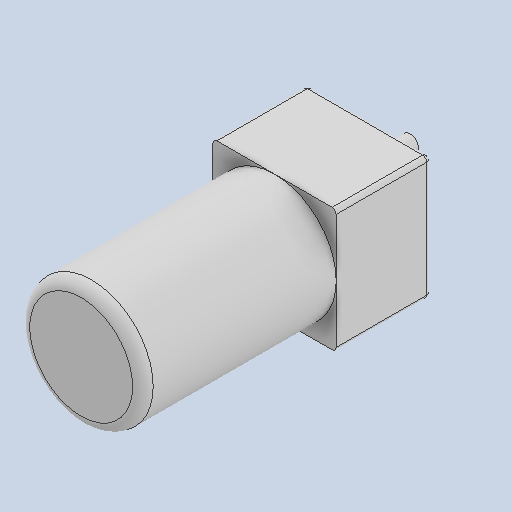
# Autodesk Inventor part: Motor
Saved by Autodesk Inventor 2026 (Build 300175050, 175E)
## iProperties
Created: 2025-11-23
Part Number: Motor
Material: Generic
Document SubType Name: Modeling
Designer: Kartik
Mass: 431.593 g
Surface Area: 359.676 cm^2
Volume: 431.593 cm^3
Density: 1 g/cm^3
Appearance: Default
Author: Kartik
Autodesk Inventor part; units mm, degrees
ref_plane "YZ Plane" through (0, 0, 0) normal (1, 0, 0) x (0, 1, 0)
ref_plane "XZ Plane" through (0, 0, 0) normal (0, 1, 0) x (-1, 0, 0)
ref_plane "XY Plane" through (0, 0, 0) normal (0, 0, 1) x (1, 0, 0)
sketch "Sketch1" plane through (0, 0, 0) normal (0, 0, 1) x (1, 0, 0)
  line L0 (-30, 30) -> (30, 30)
  line L1 (30, 30) -> (30, -30)
  line L2 (30, -30) -> (-30, -30)
  line L3 (-30, -30) -> (-30, 30)
  point P0 (0, 0)
  dimension "d0" = 60
  dimension "d1" = 60
  dimension "d2" = 30
  dimension "d3" = 30
  constraints: 8 end point, 2 parallel, 1 horizontal, 1 perpendicular
  measures "d0" distance of L0.start L0.end
  measures "d1" distance of L0.end L1.end
  measures "d2" distance from line of L1 point (0, 0)
  measures "d3" distance from line of L0 point (0, 0)
extrude "Extrusion1" add sketch "Sketch1" along normal blind 46
sketch "Sketch2" plane through (0, 0, 46) normal (0, 0, 1) x (1, 0, 0)
  circle A0 centre (0, 0) radius 30
  dimension "d14" = 60
  constraints: 1 centre point, 1 coincident
  measures "d14" diameter of A0
extrude "Extrusion2" add sketch "Sketch2" along normal blind 94
fillet "Fillet1" radius 5 1 edges at (-30, 0, 140)
fillet "Fillet2" radius 2 7 edges at (30, 30, 23) (30, -30, 23) (30, 0, 0) (-30, 30, 23) (0, 30, 0) (-30, 0, 0) (0, -30, 0)
sketch "Sketch3" plane through (0, 0, 0) normal (0, 0, -1) x (-1, 0, 0)
  line L0 (30, -30) -> (30, 28) projected
  line L1 (30, 0) -> (10, 0)
  circle A0 centre (10, 0) radius 4
  point P0 (0, 0)
  dimension "d10" = 20
  dimension "d11" = 8
  dimension "d15" = 0
  constraints: 2 end point, 1 centre point, 1 coincident, 1 horizontal, 1 point on line
  measures "d10" distance of L1.start L1.end
  measures "d11" diameter of A0
  measures "d15" vertical distance of point (0, 0) L1.end
extrude "Extrusion3" add sketch "Sketch3" along normal blind 30
equation "\"d2\" = 0.5 * d0"
equation "\"d3\" = 0.5 * d1"
body "Solid1"
